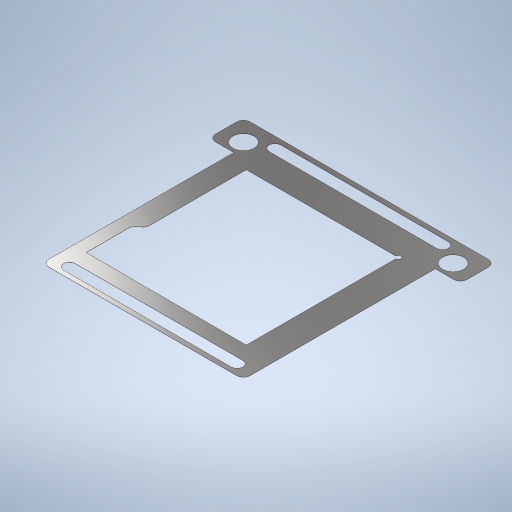
# Autodesk Inventor part: Baseplate Film Stencil - V1
Saved by Autodesk Inventor 2023 (Build 270158000, 158)
## iProperties
Created: 2022-06-23
Part Number: Baseplate Film Stencil - V1
Material: Stainless Steel
Document SubType Name: Modeling
Designer: Caleb
Density: 8 g/cm^3
Appearance: Semi-Polished
Author: Caleb
Autodesk Inventor part; units mm, degrees
ref_plane "YZ Plane" through (0, 0, 0) normal (1, 0, 0) x (0, 1, 0)
ref_plane "XZ Plane" through (0, 0, 0) normal (0, 1, 0) x (-1, 0, 0)
ref_plane "XY Plane" through (0, 0, 0) normal (0, 0, 1) x (1, 0, 0)
sketch "Sketch1" plane through (0, 0, 0) normal (0, 1, 0) x (-1, 0, 0)
  line L0 (-38.1, -34.29) -> (38.1, -34.29)
  line L1 (38.1, -34.29) -> (38.1, 34.29)
  line L2 (38.1, 34.29) -> (-38.1, 34.29)
  line L3 (-38.1, 34.29) -> (-38.1, -34.29)
  line L4 (-38.1, -34.29) -> (38.1, 34.29) construction
  line L5 (38.1, -34.29) -> (-38.1, 34.29) construction
  point P0 (0, 0)
  dimension "d0" = 76.2
  dimension "d1" = 68.58
  constraints: 12 end point, 2 midpoint, 2 parallel, 1 horizontal, 1 perpendicular
  measures "d0" distance of L2.end L1.end
  measures "d1" distance of L1.end L0.end
extrude "Extrusion1" add sketch "Sketch1" along normal blind 0.0508
sketch "Sketch2" plane through (0, 0.0508, 0) normal (0, 1, 0) x (1, 0, 0)
  line L0 (-38.1, -34.29) -> (38.1, -34.29) projected
  line L1 (-46.3971, 0) -> (43.7494, 0)
  line L2 (-38.1, 34.29) -> (-38.1, -34.29) projected
  line L3 (38.1, -34.29) -> (38.1, 34.29) projected
  line L4 (38.1, 23.79) -> (30.48, 23.79)
  line L5 (30.48, 23.79) -> (30.48, -34.29)
  line L6 (30.48, -34.29) -> (38.1, -34.29)
  line L7 (38.1, -34.29) -> (38.1, 23.79)
  line L8 (0, -45.6355) -> (0, 71.8702)
  line L9 (46.3971, 0) -> (-43.7494, 0)
  line L10 (-38.1, -34.29) -> (-38.1, 34.29)
  line L11 (-38.1, 23.79) -> (-30.48, 23.79)
  line L12 (-30.48, 23.79) -> (-30.48, -34.29)
  line L13 (-30.48, -34.29) -> (-38.1, -34.29)
  line L14 (-38.1, -34.29) -> (-38.1, 23.79)
  line L15 (38.1, 34.29) -> (-38.1, 34.29) projected
  point P0 (0, 0)
  point P1 (38.1, -27.305)
  dimension "d14" = 7.62
  dimension "d16" = 10.5
  constraints: 24 end point, 6 symmetric about line, 3 point on line, 2 horizontal, 2 parallel, 1 perpendicular, 1 vertical
  measures "d14" distance of L5.end L6.end
  measures "d16" distance between parallel lines of L15 L4
extrude "Extrusion2" cut sketch "Sketch2" against normal through all contours L2 L1 L12 L0 | L2 L11 L12 L1 | L5 L1 L3 L0 | L5 L4 L3 L1
sketch "Sketch6" plane through (0, 0.0508, 0) normal (0, 1, 0) x (1, 0, 0)
  line L0 (38.1, 34.29) -> (-38.1, 34.29) projected
  line L1 (-38.1, 34.29) -> (-38.1, 23.79) projected
  line L2 (38.1, 23.79) -> (38.1, 34.29) projected
  point P0 (0, 0)
  point P1 (-31.75, 27.94)
  point P2 (31.75, 27.94)
  point P3 (36.1, 34.29)
  point P4 (-36.1, 34.29)
  point P5 (-38.1, 32.29)
  point P6 (-38.1, 25.29)
  point P7 (38.1, 25.29)
  point P8 (38.1, 32.29)
  point P9 (38.1, 28.79)
  dimension "d41" = 6.35
  dimension "d42" = 6.35
  dimension "d43" = 6.35
  constraints: 1 horizontal alignment, 1 point on line
  measures "d41" distance from line of L0 point (-31.75, 27.94)
  measures "d42" distance from line of L1 point (-31.75, 27.94)
  measures "d43" horizontal distance of point (38.1, 28.79) point (31.75, 27.94)
hole "Hole1" at (-31.75, 0.0508, -27.94) at (31.75, 0.0508, -27.94) direction (0, -1, 0) diameter 6.3754 end through all
sketch "Sketch3" plane through (0, 0.0508, 0) normal (0, 1, 0) x (1, 0, 0)
  line L0 (25.4, -31.115) -> (-25.4, -31.115) construction
  line L1 (25.4, -29.365) -> (-25.4, -29.365)
  line L2 (-25.4, -32.865) -> (25.4, -32.865)
  arc A0 (25.4, -32.865) -> (25.4, -29.365) centre (25.4, -31.115) ccw
  arc A1 (-25.4, -29.365) -> (-25.4, -32.865) centre (-25.4, -31.115) ccw
  line L3 (25.4, 31.115) -> (-25.4, 31.115) construction
  line L4 (25.4, 32.865) -> (-25.4, 32.865)
  line L5 (-25.4, 29.365) -> (25.4, 29.365)
  arc A2 (25.4, 29.365) -> (25.4, 32.865) centre (25.4, 31.115) ccw
  arc A3 (-25.4, 32.865) -> (-25.4, 29.365) centre (-25.4, 31.115) ccw
  line L6 (38.1, 34.29) -> (-38.1, 34.29) projected
  line L7 (-38.1, -34.29) -> (38.1, -34.29) projected
  point P0 (0, 0)
  point P1 (0, -31.115)
  point P2 (0, 31.115)
  dimension "d17" = 3.5
  dimension "d18" = 3.5
  dimension "d19" = 50.8
  dimension "d20" = 50.8
  dimension "d21" = 3.175
  dimension "d22" = 3.175
  constraints: 16 end point, 8 point on circle, 8 tangent, 4 centre point, 3 parallel, 2 midpoint, 2 vertical alignment, 1 horizontal
  measures "d17" distance between parallel lines of L2 L1
  measures "d18" distance between parallel lines of L4 L5
  measures "d19" distance of L0.end L0.start
  measures "d20" distance of L3.end L3.start
  measures "d21" distance from line of L6 point (0, 31.115)
  measures "d22" distance from line of L7 point (0, -31.115)
extrude "Extrusion3" cut sketch "Sketch3" against normal through all
sketch "Sketch4" plane through (0, 0.0508, 0) normal (0, 1, 0) x (1, 0, 0)
  line L0 (-24.105, -24.825) -> (21.895, -24.825)
  line L1 (21.895, -24.825) -> (21.895, 21.175)
  line L2 (21.895, 21.175) -> (-24.105, 21.175)
  line L3 (-24.105, 21.175) -> (-24.105, -24.825)
  line L4 (38.1, 34.29) -> (-38.1, 34.29) projected
  line L5 (38.1, 23.79) -> (38.1, 34.29) projected
  circle A0 centre (21.895, 21.175) radius 0.7938
  circle A1 centre (31.75, 27.94) radius 3.1877 projected
  point P0 (0, 0)
  point P1 (21.895, 20.3813)
  point P2 (21.1012, 21.175)
  point P3 (29.845, 22.225)
  dimension "d29" = 1.5875
  dimension "d34" = 46
  dimension "d35" = 46
  dimension "d51" = 1.905
  dimension "d52" = 5.715
  dimension "d53" = 7.95
  dimension "d54" = 1.05
  constraints: 8 end point, 2 parallel, 1 centre point, 1 coincident, 1 horizontal, 1 perpendicular
  measures "d29" diameter of A0
  measures "d34" distance of L0.start L0.end
  measures "d35" distance of L2.end L0.start
  measures "d51" horizontal distance of point (29.845, 22.225) A1.centre
  measures "d52" vertical distance of point (29.845, 22.225) A1.centre
  measures "d53" distance from line of L1 point (29.845, 22.225)
  measures "d54" distance from line of L2 point (29.845, 22.225)
extrude "Extrusion4" cut sketch "Sketch4" against normal through all contours L3 L2 A0 L1 L0 | A0 L2 L1 | L1 L2 A0
sketch "Sketch5" plane through (0, 0.0508, 0) normal (0, 1, 0) x (1, 0, 0)
  line L0 (-24.105, -24.825) -> (-24.105, 21.175) projected
  line L1 (-24.105, -24.825) -> (-26.605, -24.825)
  line L2 (-26.605, -24.825) -> (-26.605, -9.825)
  line L3 (-26.605, -9.825) -> (-24.105, -9.825)
  line L4 (-24.105, -9.825) -> (-24.105, -24.825)
  point P0 (0, 0)
  point P1 (-24.105, -9.825)
  dimension "d36" = 15
  dimension "d37" = 2.5
  constraints: 8 end point, 2 parallel, 1 horizontal, 1 perpendicular
  measures "d36" distance of L1.end L2.end
  measures "d37" distance of L2.end L3.end
extrude "Extrusion5" cut sketch "Sketch5" against normal through all
fillet "Fillet2" radius 2 8 edges at (30.48, 0.0254, 34.29) (-30.48, 0.0254, 34.29) (-38.1, 0.0254, -23.79) (-38.1, 0.0254, -34.29) (38.1, 0.0254, -34.29) (38.1, 0.0254, -23.79) (-24.105, 0.0254, 9.825) (-26.605, 0.0254, 9.825)
equation "\"d42\" = d41"
equation "\"d43\" = d42"
equation "\"d18\" = d17"
equation "\"d20\" = d19"
body "Solid1"
